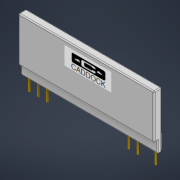
# Autodesk Inventor part: CADDOCK - HDV5 - xxxx
Saved by Autodesk Inventor 2021 (Build 250183000, 183)
## iProperties
Created: 2022-03-29
Part Number: CADDOCK - HDV5 - xxxx
Material: Generic
Document SubType Name: Modeling
Designer: Dell
Density: 1 g/cm^3
Appearance: Default
Author: Dell
Autodesk Inventor part; units mm, degrees
ref_plane "YZ Plane" through (0, 0, 0) normal (1, 0, 0) x (0, 1, 0)
ref_plane "XZ Plane" through (0, 0, 0) normal (0, 1, 0) x (-1, 0, 0)
sketch "Sketch2" plane through (0, 0, 0) normal (1, 0, 0) x (0, 1, 0)
  line L0 (0, 0) -> (-15.5, 0)
  line L1 (-15.5, 0) -> (-15.5, 2.19)
  line L2 (-15.5, 2.19) -> (0, 2.19)
  line L3 (0, 2.19) -> (0, 0)
  line L4 (23.9967, 114.2131) -> (23.9967, -36.4561) construction
  line L5 (23.9967, -36.4561) -> (-43.3153, -36.4561) construction
  line L6 (-43.3153, -36.4561) -> (-43.3153, 114.2131) construction
  line L7 (-43.3153, 114.2131) -> (23.9967, 114.2131) construction
  line L8 (-15.5, 2.19) -> (-12.516, 2.19)
  line L9 (-12.516, 2.19) -> (-12.516, 1.2565)
  line L10 (-12.516, 1.2565) -> (-15.5, 1.2565)
  line L11 (-15.5, 1.2565) -> (-15.5, 2.19)
  dimension "d7" = 15.5
  dimension "d8" = 2.19
  constraints: 16 end point, 4 parallel, 2 horizontal, 2 perpendicular, 2 other
  measures "d7" distance of L0.start L0.end
  measures "d8" distance of L2.end L0.start
extrude "Extrusion1" add sketch "Sketch2" along normal blind 38.1 contours L0 L1 L10 L9 L2 L3
ref_plane "Work Plane1" through (0, -15.5, 0.5) normal (0, 0, -1) x (-1, 0, 0)
sketch "Sketch5" plane through (0, -15.5, 0.5) normal (0, 0, -1) x (-1, 0, 0)
  line L0 (-36.1887, 45.1667) -> (-36.1887, -19.1426) construction
  line L1 (-180.1369, -19.1426) -> (-180.1369, 45.1667) construction
  line L2 (-36.1887, -19.1426) -> (-180.1369, -19.1426) construction
  line L3 (-180.1369, 45.1667) -> (-36.1887, 45.1667) construction
  line L4 (-0.8682, 0.8425) -> (-1.6718, 0.8425)
  line L5 (-1.6718, 0.8425) -> (-1.6718, -0.3212)
  line L6 (-0.8682, -0.3212) -> (-0.8682, 0.8425)
  line L7 (-1.525, -0.3212) -> (-1.525, -3.81)
  line L8 (-1.525, -3.81) -> (-1.015, -3.81)
  line L9 (-1.015, -3.81) -> (-1.015, -0.3212)
  line L10 (0, 0) -> (-38.1, 0)
  line L11 (-3.4082, 0.8425) -> (-4.2118, 0.8425)
  line L12 (-4.2118, 0.8425) -> (-4.2118, -0.3212)
  line L13 (-3.4082, -0.3212) -> (-3.4082, 0.8425)
  line L14 (-3.555, -3.81) -> (-3.555, -0.3212)
  line L15 (-4.065, -0.3212) -> (-4.065, -3.81)
  line L16 (-4.065, -3.81) -> (-3.555, -3.81)
  line L17 (-5.9482, 0.8425) -> (-6.7518, 0.8425)
  line L18 (-6.7518, 0.8425) -> (-6.7518, -0.3212)
  line L19 (-5.9482, -0.3212) -> (-5.9482, 0.8425)
  line L20 (-6.095, -3.81) -> (-6.095, -0.3212)
  line L21 (-6.605, -0.3212) -> (-6.605, -3.81)
  line L22 (-6.605, -3.81) -> (-6.095, -3.81)
  line L23 (-28.8082, 0.8425) -> (-29.6118, 0.8425)
  line L24 (-28.8082, -0.3212) -> (-28.8082, 0.8425)
  line L25 (-29.6118, 0.8425) -> (-29.6118, -0.3212)
  line L26 (-29.465, -0.3212) -> (-29.465, -3.81)
  line L27 (-28.955, -3.81) -> (-28.955, -0.3212)
  line L28 (-29.465, -3.81) -> (-28.955, -3.81)
  line L29 (-31.3482, 0.8425) -> (-32.1518, 0.8425)
  line L30 (-31.3482, -0.3212) -> (-31.3482, 0.8425)
  line L31 (-32.1518, 0.8425) -> (-32.1518, -0.3212)
  line L32 (-32.005, -0.3212) -> (-32.005, -3.81)
  line L33 (-31.495, -3.81) -> (-31.495, -0.3212)
  line L34 (-32.005, -3.81) -> (-31.495, -3.81)
  line L35 (-36.4282, 0.8425) -> (-37.2318, 0.8425)
  line L36 (-36.4282, -0.3212) -> (-36.4282, 0.8425)
  line L37 (-37.2318, 0.8425) -> (-37.2318, -0.3212)
  line L38 (-37.085, -0.3212) -> (-37.085, -3.81)
  line L39 (-36.575, -3.81) -> (-36.575, -0.3212)
  line L40 (-37.085, -3.81) -> (-36.575, -3.81)
  line L41 (-37.2318, -0.3212) -> (-37.085, -0.3212)
  line L42 (-36.575, -0.3212) -> (-36.4282, -0.3212)
  line L43 (-32.1518, -0.3212) -> (-32.005, -0.3212)
  line L44 (-31.495, -0.3212) -> (-31.3482, -0.3212)
  line L45 (-29.6118, -0.3212) -> (-29.465, -0.3212)
  line L46 (-28.955, -0.3212) -> (-28.8082, -0.3212)
  line L47 (-6.7518, -0.3212) -> (-6.605, -0.3212)
  line L48 (-6.095, -0.3212) -> (-5.9482, -0.3212)
  line L49 (-4.2118, -0.3212) -> (-4.065, -0.3212)
  line L50 (-3.555, -0.3212) -> (-3.4082, -0.3212)
  line L51 (-1.6718, -0.3212) -> (-1.525, -0.3212)
  line L52 (-1.015, -0.3212) -> (-0.8682, -0.3212)
  point P0 (0, 15.5)
  point P1 (0, 15.5)
  point P2 (-1.27, -0.3212)
  point P3 (-1.27, -3.81)
  point P4 (-3.81, -3.81)
  point P5 (-6.35, -3.81)
  point P6 (-29.21, -3.81)
  point P7 (-31.75, -3.81)
  point P8 (-36.83, -3.81)
  point P9 (-3.4082, 0)
  point P10 (-4.2118, 0)
  point P11 (-5.9482, 0)
  point P12 (-6.7518, 0)
  point P13 (-0.8682, 0)
  point P14 (-1.6718, 0)
  dimension "d141" = 3.81
  dimension "d142" = 0.51
  dimension "d143" = 1.27
  dimension "d144" = 2.54
  dimension "d145" = 2.54
  dimension "d146" = 0.51
  dimension "d147" = 0.51
  dimension "d148" = 22.86
  dimension "d149" = 2.54
  dimension "d150" = 5.08
  dimension "d151" = 0.51
  dimension "d152" = 0.51
  dimension "d153" = 0.51
  constraints: 98 end point, 24 parallel, 6 horizontal, 6 perpendicular, 1 midpoint, 2 other
  measures "d141" distance between parallel lines of L10 L8
  measures "d142" distance of L7.end L8.end
  measures "d143" horizontal distance of L10.start point (-1.27, -3.81)
  measures "d144" distance of point (-1.27, -3.81) point (-3.81, -3.81)
  measures "d145" distance of point (-3.81, -3.81) point (-6.35, -3.81)
  measures "d146" distance of L15.end L14.start
  measures "d147" distance of L21.end L20.start
  measures "d148" distance of point (-6.35, -3.81) point (-29.21, -3.81)
  measures "d149" distance of point (-29.21, -3.81) point (-31.75, -3.81)
  measures "d150" distance of point (-31.75, -3.81) point (-36.83, -3.81)
  measures "d151" distance of L26.end L27.start
  measures "d152" distance of L32.end L33.start
  measures "d153" distance of L38.end L39.start
extrude "Extrusion2" add sketch "Sketch5" along normal blind 0.25 separate body contours L36 L42 L39 L40 L38 L41 L37 L10 | L10 L37 L35 L36 | L30 L44 L33 L34 L32 L43 L31 L10 | L10 L31 L29 L30 | L24 L46 L27 L28 L26 L45 L25 L10 | L10 L25 L23 L24 | L19 L48 L20 L22 L21 L47 L18 L10 | L13 L50 L14 L16 L15 L49 L12 L10 | L6 L52 L9 L8 L7 L51 L5 L10
fillet "Fillet1" radius 0.3 14 edges at (19.05, 0, 2.19) (38.1, -6.258, 2.19) (38.1, 0, 1.095) (19.05, 0, 0) (38.1, -7.75, 0) (0, 0, 1.095) (0, -7.75, 0) (0, -6.258, 2.19) (38.1, -14.008, 1.2565) (38.1, -12.516, 1.7233) (0, -12.516, 1.7233) (19.05, -12.516, 2.19) (19.05, -15.5, 1.2565) (19.05, -15.5, 0)
sketch "Sketch6" plane through (0.3, -12.216, 2.19) normal (0, 0, 1) x (1, 0, 0)
  line L0 (12.6469, 11.0633) -> (25.8407, 11.0633) construction
  line L1 (25.8407, 11.0633) -> (25.8407, 5.9657) construction
  line L2 (25.8407, 5.9657) -> (12.6469, 5.9657) construction
  line L3 (12.6469, 5.9657) -> (12.6469, 11.0633) construction
  point P0 (-0.3, 12.216)
  constraints: 2 other
decal "Decal1"
body "Solid1"
body "Solid2"
